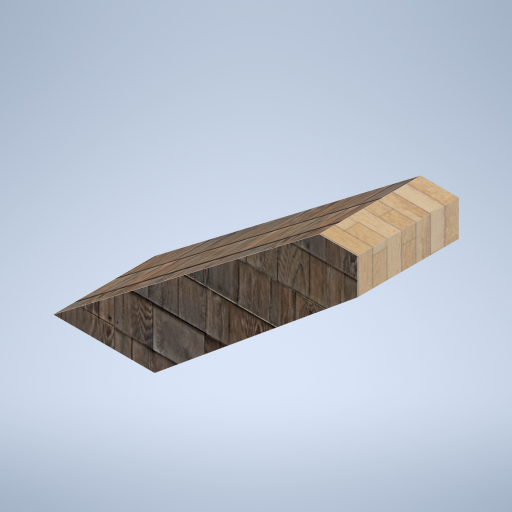
# Autodesk Inventor part: frame_rib_02
Saved by Autodesk Inventor 2024.2 (Build 282272000, 272)
## iProperties
Created: 2024-05-22
Part Number: frame_rib_02
Material: Wood (Maple)
Document SubType Name: Modeling
Designer: LOSTER_1
Density: 0.67 g/cm^3
Appearance: Natural Maple - Glossy Dark Tint
Author: LOSTER_1
Autodesk Inventor part; units mm, degrees
ref_plane "YZ Plane" through (0, 0, 0) normal (1, 0, 0) x (0, 1, 0)
ref_plane "XZ Plane" through (0, 0, 0) normal (0, 1, 0) x (-1, 0, 0)
ref_plane "XY Plane" through (0, 0, 0) normal (0, 0, 1) x (1, 0, 0)
sketch "Sketch1" plane through (0, 0, 0) normal (0, 0, 1) x (1, 0, 0)
  line L0 (-12.1607, 542.4526) -> (-262.4067, 542.4526)
  line L1 (-812.1607, -257.6855) -> (-1212.1607, -257.6855)
  line L2 (-812.1607, -559.924) -> (-812.1607, -559.1779)
  line L3 (-12.1607, 542.4526) -> (-12.1607, 400.7882)
  line L4 (-12.1607, 542.4526) -> (129.5037, 542.4526) construction
  line L5 (-12.1607, 400.7882) -> (-812.1607, -257.6855)
  line L6 (-12.1607, 542.4526) -> (-162.1607, 542.4526)
  line L7 (-162.1607, 542.4526) -> (-1212.1607, -257.6855)
  point P0 (0, 0)
  dimension "d2" = 90
  dimension "d5" = 150
  constraints: 16 end point, 1 coincident, 1 horizontal, 1 perpendicular, 1 point on line
  measures "d2" angle of L3 L4
  measures "d5" distance of L0.start L6.end
extrude "Extrusion3" add sketch "Sketch1" along normal blind 400
body "Solid3"
